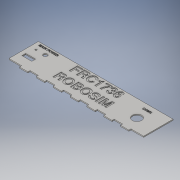
# Autodesk Inventor part: front
Saved by Autodesk Inventor 2016 (Build 200138000, 138)
## iProperties
Created: 2015-08-25
Part Number: front
Material: Generic
Document SubType Name: Modeling
Designer: Chris Gerth
Density: 1 g/cm^3
Appearance: Default
Author: Chris Gerth
Autodesk Inventor part; units mm, degrees
ref_plane "YZ Plane" through (0, 0, 0) normal (1, 0, 0) x (0, 1, 0)
ref_plane "XZ Plane" through (0, 0, 0) normal (0, 1, 0) x (-1, 0, 0)
ref_plane "XY Plane" through (0, 0, 0) normal (0, 0, 1) x (1, 0, 0)
sketch "Sketch1" plane through (0, 0, 0) normal (0, 1, 0) x (-1, 0, 0)
  line L0 (203.2, 31.75) -> (-203.2, 31.75)
  line L1 (-203.2, 31.75) -> (-203.2, -57.15)
  line L2 (-203.2, -57.15) -> (203.2, -57.15)
  line L3 (203.2, -57.15) -> (203.2, 31.75)
  point P0 (0, 0)
  dimension "d0" = 406.4
  dimension "d1" = 88.9
  constraints: 8 end point, 2 parallel, 1 horizontal, 1 perpendicular
  measures "d0" distance of L2.end L1.end
  measures "d1" distance of L1.end L0.end
extrude "Extrusion1" add sketch "Sketch1" along normal blind 3.175
sketch "Sketch2" plane through (0, 3.175, 0) normal (0, 1, 0) x (1, 0, 0)
  line L0 (-203.2, -31.75) -> (203.2, -31.75) projected
  line L1 (-165.1, -31.75) -> (-139.7, -31.75)
  line L2 (-139.7, -31.75) -> (-139.7, -38.1)
  line L3 (-139.7, -38.1) -> (-165.1, -38.1)
  line L4 (-165.1, -38.1) -> (-165.1, -31.75)
  line L5 (-114.3, -31.75) -> (-88.9, -31.75)
  line L6 (-88.9, -31.75) -> (-88.9, -38.1)
  line L7 (-88.9, -38.1) -> (-114.3, -38.1)
  line L8 (-114.3, -38.1) -> (-114.3, -31.75)
  line L9 (-63.5, -31.75) -> (-38.1, -31.75)
  line L10 (-38.1, -31.75) -> (-38.1, -38.1)
  line L11 (-38.1, -38.1) -> (-63.5, -38.1)
  line L12 (-63.5, -38.1) -> (-63.5, -31.75)
  line L13 (-12.7, -31.75) -> (12.7, -31.75)
  line L14 (12.7, -31.75) -> (12.7, -38.1)
  line L15 (12.7, -38.1) -> (-12.7, -38.1)
  line L16 (-12.7, -38.1) -> (-12.7, -31.75)
  line L17 (38.1, -31.75) -> (63.5, -31.75)
  line L18 (63.5, -31.75) -> (63.5, -38.1)
  line L19 (63.5, -38.1) -> (38.1, -38.1)
  line L20 (38.1, -38.1) -> (38.1, -31.75)
  line L21 (88.9, -31.75) -> (114.3, -31.75)
  line L22 (114.3, -31.75) -> (114.3, -38.1)
  line L23 (114.3, -38.1) -> (88.9, -38.1)
  line L24 (88.9, -38.1) -> (88.9, -31.75)
  line L25 (139.7, -31.75) -> (165.1, -31.75)
  line L26 (165.1, -31.75) -> (165.1, -38.1)
  line L27 (165.1, -38.1) -> (139.7, -38.1)
  line L28 (139.7, -38.1) -> (139.7, -31.75)
  point P0 (0, 0)
  dimension "d6" = 50.8
  constraints: 56 end point, 2 horizontal, 2 parallel, 1 collinear, 1 perpendicular, 1 point on line, 47 other
  measures "d6" distance of L1.start L5.start
extrude "Extrusion2" add sketch "Sketch2" against normal blind 3.175
sketch "Sketch3" plane through (-210.3014, 3.175, 39.6064) normal (0, 1, 0) x (1, 0, 0)
  circle A0 centre (355.6026, 45.722) radius 13.97
  point P0 (203.2, 0)
  dimension "d13" = 27.94
  constraints: 1 centre point
  measures "d13" diameter of A0
extrude "Extrusion3" cut sketch "Sketch3" against normal blind 5
sketch "Sketch4" plane through (-216.1175, 3.175, 42.2546) normal (0, 1, 0) x (1, 0, 0)
  line L0 (344.7979, 86.0656) -> (387.5444, 86.0656) construction
  line L1 (387.5444, 86.0656) -> (387.5444, 74.2339) construction
  line L2 (387.5444, 74.2339) -> (344.7979, 74.2339) construction
  line L3 (344.7979, 74.2339) -> (344.7979, 86.0656) construction
  spline S0 degree 2 poles (350.7726, 81.7796) (350.6492, 80.5846) (349.8641, 79.9773) knots 0 0 0 1 1 1
  spline S1 degree 2 poles (349.8641, 79.9773) (349.1431, 79.4193) (347.963, 79.4193) knots 0 0 0 1 1 1
  spline S2 degree 2 poles (347.963, 79.4193) (346.6742, 79.4193) (345.1781, 81.2315) (345.1781, 82.7819) knots 0 0 0 1 2 2 2
  spline S3 degree 2 poles (345.1781, 82.7819) (345.1781, 84.2188) (345.9188, 85.1175) knots 0 0 0 1 1 1
  spline S4 degree 2 poles (345.9188, 85.1175) (346.7039, 86.0656) (348.0865, 86.0656) knots 0 0 0 1 1 1
  spline S5 degree 2 poles (348.0865, 86.0656) (349.2468, 86.0656) (350.743, 84.8212) (350.7726, 83.809) knots 0 0 0 1 2 2 2
  line L4 (350.7726, 83.809) -> (349.5233, 83.809)
  spline S6 degree 2 poles (349.5233, 83.809) (349.474, 84.3126) (348.679, 84.9743) (348.126, 84.9743) knots 0 0 0 1 2 2 2
  spline S7 degree 2 poles (348.126, 84.9743) (347.3507, 84.9743) (346.452, 83.7744) (346.452, 82.7474) knots 0 0 0 1 2 2 2
  spline S8 degree 2 poles (346.452, 82.7474) (346.452, 81.7302) (347.3408, 80.5352) (348.0815, 80.5352) knots 0 0 0 1 2 2 2
  spline S9 degree 2 poles (348.0815, 80.5352) (348.6642, 80.5352) (349.4838, 81.2216) (349.5085, 81.7796) knots 0 0 0 1 2 2 2
  line L5 (349.5085, 81.7796) -> (350.7726, 81.7796)
  spline S10 degree 2 poles (357.5473, 82.7276) (357.5473, 81.2315) (355.8487, 79.4193) (354.4908, 79.4193) knots 0 0 0 1 2 2 2
  spline S11 degree 2 poles (354.4908, 79.4193) (353.0341, 79.4193) (352.2095, 80.4019) knots 0 0 0 1 1 1
  spline S12 degree 2 poles (352.2095, 80.4019) (351.4343, 81.3105) (351.4343, 82.7474) knots 0 0 0 1 1 1
  spline S13 degree 2 poles (351.4343, 82.7474) (351.4343, 84.1299) (352.1651, 85.0385) knots 0 0 0 1 1 1
  spline S14 degree 2 poles (352.1651, 85.0385) (353.0094, 86.0656) (354.5451, 86.0656) knots 0 0 0 1 1 1
  spline S15 degree 2 poles (354.5451, 86.0656) (355.9622, 86.0656) (356.7819, 85.0829) knots 0 0 0 1 1 1
  spline S16 degree 2 poles (356.7819, 85.0829) (357.5473, 84.1596) (357.5473, 82.7276) knots 0 0 0 1 1 1
  spline S17 degree 2 poles (356.2931, 82.7326) (356.2931, 83.7596) (355.3253, 84.9249) (354.471, 84.9249) knots 0 0 0 1 2 2 2
  spline S18 degree 2 poles (354.471, 84.9249) (353.6464, 84.9249) (352.6885, 83.7645) (352.6885, 82.7671) knots 0 0 0 1 2 2 2
  spline S19 degree 2 poles (352.6885, 82.7671) (352.6885, 81.7302) (353.681, 80.5451) (354.5599, 80.5451) knots 0 0 0 1 2 2 2
  spline S20 degree 2 poles (354.5599, 80.5451) (355.3351, 80.5451) (356.2931, 81.7549) (356.2931, 82.7326) knots 0 0 0 1 2 2 2
  line L6 (364.6182, 79.6119) -> (363.3097, 79.6119)
  line L7 (363.3097, 79.6119) -> (363.3097, 84.7669)
  line L8 (363.3097, 84.7669) -> (362.1838, 79.6119)
  line L9 (362.1838, 79.6119) -> (360.8753, 79.6119)
  line L10 (360.8753, 79.6119) -> (359.7446, 84.7422)
  line L11 (359.7446, 84.7422) -> (359.7446, 79.6119)
  line L12 (359.7446, 79.6119) -> (358.4361, 79.6119)
  line L13 (358.4361, 79.6119) -> (358.4361, 85.9619)
  line L14 (358.4361, 85.9619) -> (360.3519, 85.9619)
  line L15 (360.3519, 85.9619) -> (361.5271, 81.1031)
  line L16 (361.5271, 81.1031) -> (362.7171, 85.9619)
  line L17 (362.7171, 85.9619) -> (364.6182, 85.9619)
  line L18 (364.6182, 85.9619) -> (364.6182, 79.6119)
  spline S21 degree 2 poles (370.6324, 81.4833) (370.6324, 80.4908) (369.2301, 79.4094) (367.966, 79.4094) knots 0 0 0 1 2 2 2
  spline S22 degree 2 poles (367.966, 79.4094) (366.8254, 79.4094) (365.502, 80.5056) (365.3983, 81.4932) knots 0 0 0 1 2 2 2
  line L19 (365.3983, 81.4932) -> (366.6624, 81.4932)
  spline S23 degree 2 poles (366.6624, 81.4932) (366.8007, 80.4612) (368.0796, 80.4612) knots 0 0 0 1 1 1
  spline S24 degree 2 poles (368.0796, 80.4612) (368.6721, 80.4612) (369.3782, 80.9056) (369.3782, 81.2907) knots 0 0 0 1 2 2 2
  spline S25 degree 2 poles (369.3782, 81.2907) (369.3782, 81.9968) (368.4993, 82.1647) knots 0 0 0 1 1 1
  line L20 (368.4993, 82.1647) -> (366.9488, 82.461)
  spline S26 degree 2 poles (366.9488, 82.461) (366.3118, 82.5844) (365.5119, 83.4732) (365.5119, 84.0707) knots 0 0 0 1 2 2 2
  spline S27 degree 2 poles (365.5119, 84.0707) (365.5119, 85.0039) (366.7908, 86.0656) (367.9067, 86.0656) knots 0 0 0 1 2 2 2
  spline S28 degree 2 poles (367.9067, 86.0656) (369.1066, 86.0656) (370.4398, 85.0039) (370.4349, 84.0263) knots 0 0 0 1 2 2 2
  line L21 (370.4349, 84.0263) -> (369.2153, 84.0263)
  spline S29 degree 2 poles (369.2153, 84.0263) (369.1856, 84.4904) (368.4499, 85.0286) (367.8574, 85.0286) knots 0 0 0 1 2 2 2
  spline S30 degree 2 poles (367.8574, 85.0286) (366.7414, 85.0286) (366.7414, 84.2089) knots 0 0 0 1 1 1
  spline S31 degree 2 poles (366.7414, 84.2089) (366.7414, 83.6806) (367.4969, 83.5226) knots 0 0 0 1 1 1
  line L22 (367.4969, 83.5226) -> (368.84, 83.2461)
  spline S32 degree 2 poles (368.84, 83.2461) (369.7535, 83.0535) (370.1436, 82.7227) knots 0 0 0 1 1 1
  spline S33 degree 2 poles (370.1436, 82.7227) (370.6324, 82.303) (370.6324, 81.4833) knots 0 0 0 1 1 1
  point P0 (203.2, 0)
  constraints: 2 other
extrude "Extrusion4" cut sketch "Sketch4" against normal blind 1.905
sketch "Sketch5" plane through (-208.4957, 3.175, 40.5353) normal (0, 1, 0) x (1, 0, 0)
  line L0 (17.4181, 47.0558) -> (47.4181, 47.0558)
  line L1 (47.4181, 47.0558) -> (47.4181, 35.5558)
  line L2 (47.4181, 35.5558) -> (17.4181, 35.5558)
  line L3 (17.4181, 35.5558) -> (17.4181, 47.0558)
  point P0 (203.2, 0)
  dimension "d21" = 30
  dimension "d22" = 11.5
  constraints: 8 end point, 2 parallel, 1 horizontal, 1 perpendicular
  measures "d21" distance of L1.end L2.end
  measures "d22" distance of L0.end L1.end
extrude "Extrusion5" cut sketch "Sketch5" against normal blind 5
sketch "Sketch6" plane through (-204.3689, 3.175, 34.8523) normal (0, 1, 0) x (1, 0, 0)
  circle A0 centre (19.1442, 66.6446) radius 2.5
  circle A1 centre (47.3951, 66.6446) radius 6
  point P0 (203.2, 0)
  dimension "d28" = 5
  dimension "d27" = 12
  constraints: 2 centre point
  measures "d28" diameter of A0
  measures "d27" diameter of A1
extrude "Extrusion6" cut sketch "Sketch6" against normal blind 5
sketch "Sketch7" plane through (-201.7656, 3.175, 34.3855) normal (0, 1, 0) x (1, 0, 0)
  line L0 (8.5764, 86.8624) -> (71.354, 86.8624) construction
  line L1 (71.354, 86.8624) -> (71.354, 63.658) construction
  line L2 (71.354, 63.658) -> (8.5764, 63.658) construction
  line L3 (8.5764, 63.658) -> (8.5764, 86.8624) construction
  line L4 (15.3313, 80.4087) -> (14.0227, 80.4087)
  line L5 (14.0227, 80.4087) -> (14.0227, 85.5637)
  line L6 (14.0227, 85.5637) -> (12.8969, 80.4087)
  line L7 (12.8969, 80.4087) -> (11.5884, 80.4087)
  line L8 (11.5884, 80.4087) -> (10.4577, 85.539)
  line L9 (10.4577, 85.539) -> (10.4577, 80.4087)
  line L10 (10.4577, 80.4087) -> (9.1491, 80.4087)
  line L11 (9.1491, 80.4087) -> (9.1491, 86.7587)
  line L12 (9.1491, 86.7587) -> (11.065, 86.7587)
  line L13 (11.065, 86.7587) -> (12.2402, 81.8999)
  line L14 (12.2402, 81.8999) -> (13.4302, 86.7587)
  line L15 (13.4302, 86.7587) -> (15.3313, 86.7587)
  line L16 (15.3313, 86.7587) -> (15.3313, 80.4087)
  line L17 (21.9528, 80.4087) -> (20.6246, 80.4087)
  line L18 (20.6246, 80.4087) -> (20.1752, 81.6826)
  line L19 (20.1752, 81.6826) -> (17.8248, 81.6826)
  line L20 (17.8248, 81.6826) -> (17.3903, 80.4087)
  line L21 (17.3903, 80.4087) -> (16.0571, 80.4087)
  line L22 (16.0571, 80.4087) -> (18.2692, 86.7587)
  line L23 (18.2692, 86.7587) -> (19.7753, 86.7587)
  line L24 (19.7753, 86.7587) -> (21.9528, 80.4087)
  line L25 (19.8642, 82.7739) -> (19.0297, 85.2428)
  line L26 (19.0297, 85.2428) -> (18.2446, 82.7739)
  line L27 (18.2446, 82.7739) -> (19.8642, 82.7739)
  line L28 (23.9823, 80.4087) -> (22.6738, 80.4087)
  line L29 (22.6738, 80.4087) -> (22.6738, 86.7587)
  line L30 (22.6738, 86.7587) -> (23.9823, 86.7587)
  line L31 (23.9823, 86.7587) -> (23.9823, 80.4087)
  line L32 (30.2977, 80.4087) -> (29.0089, 80.4087)
  line L33 (29.0089, 80.4087) -> (26.4413, 84.8477)
  line L34 (26.4413, 84.8477) -> (26.4413, 80.4087)
  line L35 (26.4413, 80.4087) -> (25.1328, 80.4087)
  line L36 (25.1328, 80.4087) -> (25.1328, 86.7587)
  line L37 (25.1328, 86.7587) -> (26.4215, 86.7587)
  line L38 (26.4215, 86.7587) -> (28.9892, 82.4035)
  line L39 (28.9892, 82.4035) -> (28.9892, 86.7587)
  line L40 (28.9892, 86.7587) -> (30.2977, 86.7587)
  line L41 (30.2977, 86.7587) -> (30.2977, 80.4087)
  spline S0 degree 2 poles (38.766, 84.7292) (38.766, 83.8503) (37.7192, 82.6751) (37.0427, 82.6751) knots 0 0 0 1 2 2 2
  line L42 (37.0427, 82.6751) -> (35.2207, 82.6751)
  line L43 (35.2207, 82.6751) -> (35.2207, 80.4087)
  line L44 (35.2207, 80.4087) -> (33.9122, 80.4087)
  line L45 (33.9122, 80.4087) -> (33.9122, 86.7587)
  line L46 (33.9122, 86.7587) -> (36.8995, 86.7587)
  spline S1 degree 2 poles (36.8995, 86.7587) (37.8229, 86.7587) (38.766, 85.6773) (38.766, 84.7292) knots 0 0 0 1 2 2 2
  spline S2 degree 2 poles (37.5019, 84.8082) (37.5019, 85.1983) (37.0822, 85.6674) (36.7119, 85.6674) knots 0 0 0 1 2 2 2
  line L47 (36.7119, 85.6674) -> (35.2207, 85.6674)
  line L48 (35.2207, 85.6674) -> (35.2207, 83.7664)
  line L49 (35.2207, 83.7664) -> (36.7465, 83.7664)
  spline S3 degree 2 poles (36.7465, 83.7664) (37.0575, 83.7664) (37.2847, 84.1071) knots 0 0 0 1 1 1
  spline S4 degree 2 poles (37.2847, 84.1071) (37.5019, 84.4181) (37.5019, 84.8082) knots 0 0 0 1 1 1
  spline S5 degree 2 poles (45.5209, 83.5244) (45.5209, 82.0283) (43.8223, 80.2161) (42.4644, 80.2161) knots 0 0 0 1 2 2 2
  spline S6 degree 2 poles (42.4644, 80.2161) (41.0078, 80.2161) (40.1832, 81.1987) knots 0 0 0 1 1 1
  spline S7 degree 2 poles (40.1832, 81.1987) (39.4079, 82.1073) (39.4079, 83.5442) knots 0 0 0 1 1 1
  spline S8 degree 2 poles (39.4079, 83.5442) (39.4079, 84.9267) (40.1387, 85.8353) knots 0 0 0 1 1 1
  spline S9 degree 2 poles (40.1387, 85.8353) (40.9831, 86.8624) (42.5187, 86.8624) knots 0 0 0 1 1 1
  spline S10 degree 2 poles (42.5187, 86.8624) (43.9359, 86.8624) (44.7556, 85.8797) knots 0 0 0 1 1 1
  spline S11 degree 2 poles (44.7556, 85.8797) (45.5209, 84.9564) (45.5209, 83.5244) knots 0 0 0 1 1 1
  spline S12 degree 2 poles (44.2667, 83.5293) (44.2667, 84.5564) (43.2989, 85.7217) (42.4447, 85.7217) knots 0 0 0 1 2 2 2
  spline S13 degree 2 poles (42.4447, 85.7217) (41.6201, 85.7217) (40.6621, 84.5613) (40.6621, 83.5639) knots 0 0 0 1 2 2 2
  spline S14 degree 2 poles (40.6621, 83.5639) (40.6621, 82.527) (41.6546, 81.3419) (42.5336, 81.3419) knots 0 0 0 1 2 2 2
  spline S15 degree 2 poles (42.5336, 81.3419) (43.3088, 81.3419) (44.2667, 82.5517) (44.2667, 83.5293) knots 0 0 0 1 2 2 2
  line L50 (53.9547, 86.7587) -> (52.1771, 80.4087)
  line L51 (52.1771, 80.4087) -> (51.0019, 80.4087)
  line L52 (51.0019, 80.4087) -> (49.9501, 85.2526)
  line L53 (49.9501, 85.2526) -> (48.9033, 80.4087)
  line L54 (48.9033, 80.4087) -> (47.7281, 80.4087)
  line L55 (47.7281, 80.4087) -> (45.9505, 86.7587)
  line L56 (45.9505, 86.7587) -> (47.3331, 86.7587)
  line L57 (47.3331, 86.7587) -> (48.3108, 82.0036)
  line L58 (48.3108, 82.0036) -> (49.2588, 86.7587)
  line L59 (49.2588, 86.7587) -> (50.6463, 86.7587)
  line L60 (50.6463, 86.7587) -> (51.5944, 81.9493)
  line L61 (51.5944, 81.9493) -> (52.5721, 86.7587)
  line L62 (52.5721, 86.7587) -> (53.9547, 86.7587)
  line L63 (59.4899, 80.4087) -> (54.7447, 80.4087)
  line L64 (54.7447, 80.4087) -> (54.7447, 86.7587)
  line L65 (54.7447, 86.7587) -> (59.3418, 86.7587)
  line L66 (59.3418, 86.7587) -> (59.3418, 85.6674)
  line L67 (59.3418, 85.6674) -> (56.0532, 85.6674)
  line L68 (56.0532, 85.6674) -> (56.0532, 84.2256)
  line L69 (56.0532, 84.2256) -> (59.09, 84.2256)
  line L70 (59.09, 84.2256) -> (59.09, 83.1343)
  line L71 (59.09, 83.1343) -> (56.0532, 83.1343)
  line L72 (56.0532, 83.1343) -> (56.0532, 81.4999)
  line L73 (56.0532, 81.4999) -> (59.4899, 81.4999)
  line L74 (59.4899, 81.4999) -> (59.4899, 80.4087)
  line L75 (65.7659, 80.4087) -> (64.3537, 80.4087)
  spline S16 degree 2 poles (64.3537, 80.4087) (64.1808, 80.8629) (64.1808, 81.1395) knots 0 0 0 1 1 1
  line L76 (64.1808, 81.1395) -> (64.1808, 82.0974)
  spline S17 degree 2 poles (64.1808, 82.0974) (64.1808, 82.4825) (64.0673, 82.6554) knots 0 0 0 1 1 1
  spline S18 degree 2 poles (64.0673, 82.6554) (63.9043, 82.9171) (63.4253, 82.9171) knots 0 0 0 1 1 1
  line L77 (63.4253, 82.9171) -> (61.8749, 82.9171)
  line L78 (61.8749, 82.9171) -> (61.8749, 80.4087)
  line L79 (61.8749, 80.4087) -> (60.5664, 80.4087)
  line L80 (60.5664, 80.4087) -> (60.5664, 86.7587)
  line L81 (60.5664, 86.7587) -> (64.1364, 86.7587)
  spline S19 degree 2 poles (64.1364, 86.7587) (64.7289, 86.7587) (65.1635, 86.3587) knots 0 0 0 1 1 1
  spline S20 degree 2 poles (65.1635, 86.3587) (65.6967, 85.8797) (65.6967, 85.0008) knots 0 0 0 1 1 1
  spline S21 degree 2 poles (65.6967, 85.0008) (65.6967, 83.9787) (64.7635, 83.4652) knots 0 0 0 1 1 1
  spline S22 degree 2 poles (64.7635, 83.4652) (65.44, 83.0998) (65.4597, 82.6455) knots 0 0 0 1 1 1
  line L82 (65.4597, 82.6455) -> (65.5288, 81.095)
  spline S23 degree 2 poles (65.5288, 81.095) (65.5387, 80.8086) (65.7659, 80.6506) knots 0 0 0 1 1 1
  line L83 (65.7659, 80.6506) -> (65.7659, 80.4087)
  spline S24 degree 2 poles (64.4524, 84.9218) (64.4524, 85.6674) (63.7019, 85.6674) knots 0 0 0 1 1 1
  line L84 (63.7019, 85.6674) -> (61.8749, 85.6674)
  line L85 (61.8749, 85.6674) -> (61.8749, 84.0083)
  line L86 (61.8749, 84.0083) -> (63.6772, 84.0083)
  spline S25 degree 2 poles (63.6772, 84.0083) (63.9734, 84.0083) (64.4524, 84.5811) (64.4524, 84.9218) knots 0 0 0 1 2 2 2
  point P0 (203.2, 0)
  constraints: 2 other
extrude "Extrusion7" cut sketch "Sketch7" against normal blind 1.905
sketch "Sketch8" plane through (-218.0152, 3.175, 33.7162) normal (0, 1, 0) x (1, 0, 0)
  line L0 (67.968, 86.6448) -> (350.6513, 86.6448) construction
  line L1 (350.6513, 86.6448) -> (350.6513, 3.4424) construction
  line L2 (350.6513, 3.4424) -> (67.968, 3.4424) construction
  line L3 (67.968, 3.4424) -> (67.968, 86.6448) construction
  line L4 (155.152, 81.865) -> (142.5507, 81.865)
  line L5 (142.5507, 81.865) -> (142.5507, 76.0977)
  line L6 (142.5507, 76.0977) -> (153.6509, 76.0977)
  line L7 (153.6509, 76.0977) -> (153.6509, 71.7326)
  line L8 (153.6509, 71.7326) -> (142.5507, 71.7326)
  line L9 (142.5507, 71.7326) -> (142.5507, 60.83)
  line L10 (142.5507, 60.83) -> (137.3167, 60.83)
  line L11 (137.3167, 60.83) -> (137.3167, 86.23)
  line L12 (137.3167, 86.23) -> (155.152, 86.23)
  line L13 (155.152, 86.23) -> (155.152, 81.865)
  line L14 (179.6237, 60.83) -> (173.9748, 60.83)
  spline S0 degree 2 poles (173.9748, 60.83) (173.2835, 62.6471) (173.2835, 63.7532) knots 0 0 0 1 1 1
  line L15 (173.2835, 63.7532) -> (173.2835, 67.5849)
  spline S1 degree 2 poles (173.2835, 67.5849) (173.2835, 69.1255) (172.8293, 69.8168) knots 0 0 0 1 1 1
  spline S2 degree 2 poles (172.8293, 69.8168) (172.1775, 70.8636) (170.2616, 70.8636) knots 0 0 0 1 1 1
  line L16 (170.2616, 70.8636) -> (164.0597, 70.8636)
  line L17 (164.0597, 70.8636) -> (164.0597, 60.83)
  line L18 (164.0597, 60.83) -> (158.8257, 60.83)
  line L19 (158.8257, 60.83) -> (158.8257, 86.23)
  line L20 (158.8257, 86.23) -> (173.1058, 86.23)
  spline S3 degree 2 poles (173.1058, 86.23) (175.4759, 86.23) (177.214, 84.6302) knots 0 0 0 1 1 1
  spline S4 degree 2 poles (177.214, 84.6302) (179.3471, 82.7143) (179.3471, 79.1986) knots 0 0 0 1 1 1
  spline S5 degree 2 poles (179.3471, 79.1986) (179.3471, 75.1101) (175.6142, 73.056) knots 0 0 0 1 1 1
  spline S6 degree 2 poles (175.6142, 73.056) (178.3201, 71.5944) (178.3991, 69.7773) knots 0 0 0 1 1 1
  line L21 (178.3991, 69.7773) -> (178.6756, 63.5754)
  spline S7 degree 2 poles (178.6756, 63.5754) (178.7151, 62.4298) (179.6237, 61.7978) knots 0 0 0 1 1 1
  line L22 (179.6237, 61.7978) -> (179.6237, 60.83)
  spline S8 degree 2 poles (174.3699, 78.8826) (174.3699, 81.865) (171.3677, 81.865) knots 0 0 0 1 1 1
  line L23 (171.3677, 81.865) -> (164.0597, 81.865)
  line L24 (164.0597, 81.865) -> (164.0597, 75.2286)
  line L25 (164.0597, 75.2286) -> (171.2689, 75.2286)
  spline S9 degree 2 poles (171.2689, 75.2286) (172.454, 75.2286) (174.3699, 77.5197) (174.3699, 78.8826) knots 0 0 0 1 2 2 2
  spline S10 degree 2 poles (205.1027, 69.5008) (204.6089, 64.721) (201.4685, 62.2916) knots 0 0 0 1 1 1
  spline S11 degree 2 poles (201.4685, 62.2916) (198.5848, 60.0597) (193.8643, 60.0597) knots 0 0 0 1 1 1
  spline S12 degree 2 poles (193.8643, 60.0597) (188.7092, 60.0597) (182.7246, 67.3084) (182.7246, 73.5103) knots 0 0 0 1 2 2 2
  spline S13 degree 2 poles (182.7246, 73.5103) (182.7246, 79.2578) (185.6873, 82.8526) knots 0 0 0 1 1 1
  spline S14 degree 2 poles (185.6873, 82.8526) (188.8277, 86.6448) (194.358, 86.6448) knots 0 0 0 1 1 1
  spline S15 degree 2 poles (194.358, 86.6448) (198.9996, 86.6448) (204.9842, 81.6675) (205.1027, 77.6185) knots 0 0 0 1 2 2 2
  line L26 (205.1027, 77.6185) -> (200.1056, 77.6185)
  spline S16 degree 2 poles (200.1056, 77.6185) (199.9081, 79.6331) (196.7282, 82.2798) (194.516, 82.2798) knots 0 0 0 1 2 2 2
  spline S17 degree 2 poles (194.516, 82.2798) (191.4151, 82.2798) (187.8204, 77.4802) (187.8204, 73.372) knots 0 0 0 1 2 2 2
  spline S18 degree 2 poles (187.8204, 73.372) (187.8204, 69.3033) (191.3756, 64.5235) (194.3383, 64.5235) knots 0 0 0 1 2 2 2
  spline S19 degree 2 poles (194.3383, 64.5235) (196.6689, 64.5235) (199.9476, 67.2689) (200.0464, 69.5008) knots 0 0 0 1 2 2 2
  line L27 (200.0464, 69.5008) -> (205.1027, 69.5008)
  line L28 (219.5605, 60.83) -> (214.682, 60.83)
  line L29 (214.682, 60.83) -> (214.682, 77.895)
  line L30 (214.682, 77.895) -> (208.7566, 77.895)
  line L31 (208.7566, 77.895) -> (208.7566, 81.0749)
  spline S20 degree 2 poles (208.7566, 81.0749) (212.2723, 81.4305) (213.7734, 82.2008) knots 0 0 0 1 1 1
  spline S21 degree 2 poles (213.7734, 82.2008) (215.5115, 83.1291) (216.4596, 85.5387) knots 0 0 0 1 1 1
  line L32 (216.4596, 85.5387) -> (219.5605, 85.5387)
  line L33 (219.5605, 85.5387) -> (219.5605, 60.83)
  spline S22 degree 2 poles (244.131, 81.8057) (237.9291, 74.083) (236.2898, 67.5256) knots 0 0 0 1 1 1
  spline S23 degree 2 poles (236.2898, 67.5256) (235.638, 64.879) (235.2429, 60.83) knots 0 0 0 1 1 1
  line L34 (235.2429, 60.83) -> (230.2657, 60.83)
  spline S24 degree 2 poles (230.2657, 60.83) (231.5495, 68.4935) (234.6504, 75.5051) (238.9364, 81.154) knots 0 0 0 1 2 2 2
  line L35 (238.9364, 81.154) -> (226.7499, 81.154)
  line L36 (226.7499, 81.154) -> (226.7499, 85.5387)
  line L37 (226.7499, 85.5387) -> (244.131, 85.5387)
  line L38 (244.131, 85.5387) -> (244.131, 81.8057)
  spline S25 degree 2 poles (263.1513, 67.9009) (263.1513, 64.2865) (258.4111, 60.0005) (254.4411, 60.0005) knots 0 0 0 1 2 2 2
  spline S26 degree 2 poles (254.4411, 60.0005) (251.1229, 60.0005) (248.891, 61.7386) knots 0 0 0 1 1 1
  spline S27 degree 2 poles (248.891, 61.7386) (246.1456, 63.8914) (246.1456, 68.0787) knots 0 0 0 1 1 1
  line L39 (246.1456, 68.0787) -> (250.8859, 68.0787)
  spline S28 degree 2 poles (250.8859, 68.0787) (250.7081, 65.9258) (252.1499, 64.7802) knots 0 0 0 1 1 1
  spline S29 degree 2 poles (252.1499, 64.7802) (253.256, 63.8717) (254.8559, 63.8717) knots 0 0 0 1 1 1
  spline S30 degree 2 poles (254.8559, 63.8717) (256.1594, 63.8717) (258.2136, 66.5578) (258.2136, 68.0589) knots 0 0 0 1 2 2 2
  spline S31 degree 2 poles (258.2136, 68.0589) (258.2136, 69.955) (255.2509, 72.0289) (252.703, 71.9104) knots 0 0 0 1 2 2 2
  line L40 (252.703, 71.9104) -> (252.703, 75.2286)
  spline S32 degree 2 poles (252.703, 75.2286) (257.6408, 75.0903) (257.6408, 78.9813) knots 0 0 0 1 1 1
  spline S33 degree 2 poles (257.6408, 78.9813) (257.6408, 82.2205) (254.2238, 82.2205) knots 0 0 0 1 1 1
  spline S34 degree 2 poles (254.2238, 82.2205) (252.703, 82.2205) (251.9919, 81.4502) knots 0 0 0 1 1 1
  spline S35 degree 2 poles (251.9919, 81.4502) (251.0834, 80.4429) (250.9846, 77.7568) knots 0 0 0 1 1 1
  line L41 (250.9846, 77.7568) -> (246.5209, 77.7568)
  spline S36 degree 2 poles (246.5209, 77.7568) (246.4616, 78.3098) (246.4616, 78.8431) knots 0 0 0 1 1 1
  spline S37 degree 2 poles (246.4616, 78.8431) (246.4616, 82.0428) (251.0241, 86.0917) (254.5003, 86.0917) knots 0 0 0 1 2 2 2
  spline S38 degree 2 poles (254.5003, 86.0917) (257.9963, 86.0917) (260.0702, 84.4524) knots 0 0 0 1 1 1
  spline S39 degree 2 poles (260.0702, 84.4524) (262.3415, 82.7143) (262.3415, 79.4751) knots 0 0 0 1 1 1
  spline S40 degree 2 poles (262.3415, 79.4751) (262.3415, 77.5987) (261.7095, 76.4334) knots 0 0 0 1 1 1
  spline S41 degree 2 poles (261.7095, 76.4334) (261.196, 75.5446) (259.6356, 74.083) knots 0 0 0 1 1 1
  spline S42 degree 2 poles (259.6356, 74.083) (263.1513, 71.8116) (263.1513, 67.9009) knots 0 0 0 1 1 1
  spline S43 degree 2 poles (282.547, 69.0267) (282.547, 65.0765) (280.3151, 62.5681) knots 0 0 0 1 1 1
  spline S44 degree 2 poles (280.3151, 62.5681) (277.9845, 60.0005) (274.1132, 60.0005) knots 0 0 0 1 1 1
  spline S45 degree 2 poles (274.1132, 60.0005) (268.7804, 60.0005) (266.8646, 64.9382) knots 0 0 0 1 1 1
  spline S46 degree 2 poles (266.8646, 64.9382) (265.6202, 68.1577) (265.6202, 74.5966) knots 0 0 0 1 1 1
  spline S47 degree 2 poles (265.6202, 74.5966) (265.6202, 79.5344) (267.9114, 82.7143) knots 0 0 0 1 1 1
  spline S48 degree 2 poles (267.9114, 82.7143) (270.3605, 86.0917) (274.5478, 86.0917) knots 0 0 0 1 1 1
  spline S49 degree 2 poles (274.5478, 86.0917) (277.8067, 86.0917) (281.9347, 82.7933) (282.1322, 79.9294) knots 0 0 0 1 2 2 2
  line L42 (282.1322, 79.9294) -> (277.6487, 79.9294)
  spline S50 degree 2 poles (277.6487, 79.9294) (276.7994, 82.181) (274.3305, 82.181) knots 0 0 0 1 1 1
  spline S51 degree 2 poles (274.3305, 82.181) (272.5529, 82.181) (270.3605, 79.2973) (270.3605, 76.9667) knots 0 0 0 1 2 2 2
  spline S52 degree 2 poles (270.3605, 76.9667) (270.3605, 76.1569) (270.4988, 75.2879) knots 0 0 0 1 1 1
  spline S53 degree 2 poles (270.4988, 75.2879) (272.7307, 77.2037) (274.7848, 77.2037) knots 0 0 0 1 1 1
  spline S54 degree 2 poles (274.7848, 77.2037) (278.3992, 77.2037) (282.547, 73.0165) (282.547, 69.0267) knots 0 0 0 1 2 2 2
  spline S55 degree 2 poles (277.945, 69.165) (277.945, 71.1796) (276.0489, 73.4115) (274.3898, 73.4115) knots 0 0 0 1 2 2 2
  spline S56 degree 2 poles (274.3898, 73.4115) (272.6714, 73.4115) (270.3605, 70.7253) (270.3605, 68.4935) knots 0 0 0 1 2 2 2
  spline S57 degree 2 poles (270.3605, 68.4935) (270.3605, 66.6566) (272.4541, 64.1087) (274.0145, 64.1087) knots 0 0 0 1 2 2 2
  spline S58 degree 2 poles (274.0145, 64.1087) (275.8118, 64.1087) (277.945, 66.8936) (277.945, 69.165) knots 0 0 0 1 2 2 2
  line L43 (149.6611, 19.9611) -> (144.0123, 19.9611)
  spline S59 degree 2 poles (144.0123, 19.9611) (143.321, 21.7782) (143.321, 22.8843) knots 0 0 0 1 1 1
  line L44 (143.321, 22.8843) -> (143.321, 26.716)
  spline S60 degree 2 poles (143.321, 26.716) (143.321, 28.2566) (142.8667, 28.9479) knots 0 0 0 1 1 1
  spline S61 degree 2 poles (142.8667, 28.9479) (142.215, 29.9947) (140.2991, 29.9947) knots 0 0 0 1 1 1
  line L45 (140.2991, 29.9947) -> (134.0972, 29.9947)
  line L46 (134.0972, 29.9947) -> (134.0972, 19.9611)
  line L47 (134.0972, 19.9611) -> (128.8632, 19.9611)
  line L48 (128.8632, 19.9611) -> (128.8632, 45.3611)
  line L49 (128.8632, 45.3611) -> (143.1433, 45.3611)
  spline S62 degree 2 poles (143.1433, 45.3611) (145.5134, 45.3611) (147.2515, 43.7613) knots 0 0 0 1 1 1
  spline S63 degree 2 poles (147.2515, 43.7613) (149.3846, 41.8454) (149.3846, 38.3297) knots 0 0 0 1 1 1
  spline S64 degree 2 poles (149.3846, 38.3297) (149.3846, 34.2412) (145.6517, 32.1871) knots 0 0 0 1 1 1
  spline S65 degree 2 poles (145.6517, 32.1871) (148.3576, 30.7255) (148.4366, 28.9084) knots 0 0 0 1 1 1
  line L50 (148.4366, 28.9084) -> (148.7131, 22.7065)
  spline S66 degree 2 poles (148.7131, 22.7065) (148.7526, 21.5609) (149.6611, 20.9289) knots 0 0 0 1 1 1
  line L51 (149.6611, 20.9289) -> (149.6611, 19.9611)
  spline S67 degree 2 poles (144.4073, 38.0137) (144.4073, 40.9961) (141.4052, 40.9961) knots 0 0 0 1 1 1
  line L52 (141.4052, 40.9961) -> (134.0972, 40.9961)
  line L53 (134.0972, 40.9961) -> (134.0972, 34.3597)
  line L54 (134.0972, 34.3597) -> (141.3064, 34.3597)
  spline S68 degree 2 poles (141.3064, 34.3597) (142.4915, 34.3597) (144.4073, 36.6508) (144.4073, 38.0137) knots 0 0 0 1 2 2 2
  spline S69 degree 2 poles (177.0758, 32.4241) (177.0758, 26.4395) (170.2814, 19.1908) (164.8498, 19.1908) knots 0 0 0 1 2 2 2
  spline S70 degree 2 poles (164.8498, 19.1908) (159.0232, 19.1908) (155.7248, 23.1213) knots 0 0 0 1 1 1
  spline S71 degree 2 poles (155.7248, 23.1213) (152.6238, 26.7555) (152.6238, 32.5031) knots 0 0 0 1 1 1
  spline S72 degree 2 poles (152.6238, 32.5031) (152.6238, 38.0334) (155.547, 41.6676) knots 0 0 0 1 1 1
  spline S73 degree 2 poles (155.547, 41.6676) (158.9244, 45.7759) (165.0671, 45.7759) knots 0 0 0 1 1 1
  spline S74 degree 2 poles (165.0671, 45.7759) (170.7356, 45.7759) (174.0143, 41.8454) knots 0 0 0 1 1 1
  spline S75 degree 2 poles (174.0143, 41.8454) (177.0758, 38.1519) (177.0758, 32.4241) knots 0 0 0 1 1 1
  spline S76 degree 2 poles (172.059, 32.4438) (172.059, 36.5521) (168.1877, 41.2134) (164.7708, 41.2134) knots 0 0 0 1 2 2 2
  spline S77 degree 2 poles (164.7708, 41.2134) (161.4723, 41.2134) (157.6406, 36.5718) (157.6406, 32.5821) knots 0 0 0 1 2 2 2
  spline S78 degree 2 poles (157.6406, 32.5821) (157.6406, 28.4344) (161.6106, 23.6941) (165.1263, 23.6941) knots 0 0 0 1 2 2 2
  spline S79 degree 2 poles (165.1263, 23.6941) (168.2272, 23.6941) (172.059, 28.5331) (172.059, 32.4438) knots 0 0 0 1 2 2 2
  spline S80 degree 2 poles (201.4882, 27.3085) (201.4882, 24.2866) (199.4341, 22.2522) knots 0 0 0 1 1 1
  spline S81 degree 2 poles (199.4341, 22.2522) (197.1034, 19.9611) (192.9162, 19.9611) knots 0 0 0 1 1 1
  line L55 (192.9162, 19.9611) -> (181.184, 19.9611)
  line L56 (181.184, 19.9611) -> (181.184, 45.3611)
  line L57 (181.184, 45.3611) -> (192.1854, 45.3611)
  spline S82 degree 2 poles (192.1854, 45.3611) (195.8591, 45.3611) (200.8364, 41.8059) (200.8364, 38.7445) knots 0 0 0 1 2 2 2
  spline S83 degree 2 poles (200.8364, 38.7445) (200.8364, 35.8213) (198.4268, 33.5104) knots 0 0 0 1 1 1
  spline S84 degree 2 poles (198.4268, 33.5104) (201.4882, 31.081) (201.4882, 27.3085) knots 0 0 0 1 1 1
  spline S85 degree 2 poles (196.5109, 27.9011) (196.5109, 30.9033) (193.094, 30.9033) knots 0 0 0 1 1 1
  line L58 (193.094, 30.9033) -> (186.4181, 30.9033)
  line L59 (186.4181, 30.9033) -> (186.4181, 24.3261)
  line L60 (186.4181, 24.3261) -> (193.094, 24.3261)
  spline S86 degree 2 poles (193.094, 24.3261) (196.5109, 24.3261) (196.5109, 27.9011) knots 0 0 0 1 1 1
  spline S87 degree 2 poles (195.8591, 38.1914) (195.8591, 40.9763) (192.6199, 40.9763) knots 0 0 0 1 1 1
  line L61 (192.6199, 40.9763) -> (186.4181, 40.9763)
  line L62 (186.4181, 40.9763) -> (186.4181, 35.2288)
  line L63 (186.4181, 35.2288) -> (192.4817, 35.2288)
  spline S88 degree 2 poles (192.4817, 35.2288) (195.8591, 35.2288) (195.8591, 38.1914) knots 0 0 0 1 1 1
  spline S89 degree 2 poles (229.3374, 32.4241) (229.3374, 26.4395) (222.5429, 19.1908) (217.1114, 19.1908) knots 0 0 0 1 2 2 2
  spline S90 degree 2 poles (217.1114, 19.1908) (211.2848, 19.1908) (207.9863, 23.1213) knots 0 0 0 1 1 1
  spline S91 degree 2 poles (207.9863, 23.1213) (204.8854, 26.7555) (204.8854, 32.5031) knots 0 0 0 1 1 1
  spline S92 degree 2 poles (204.8854, 32.5031) (204.8854, 38.0334) (207.8086, 41.6676) knots 0 0 0 1 1 1
  spline S93 degree 2 poles (207.8086, 41.6676) (211.186, 45.7759) (217.3286, 45.7759) knots 0 0 0 1 1 1
  spline S94 degree 2 poles (217.3286, 45.7759) (222.9972, 45.7759) (226.2759, 41.8454) knots 0 0 0 1 1 1
  spline S95 degree 2 poles (226.2759, 41.8454) (229.3374, 38.1519) (229.3374, 32.4241) knots 0 0 0 1 1 1
  spline S96 degree 2 poles (224.3206, 32.4438) (224.3206, 36.5521) (220.4493, 41.2134) (217.0324, 41.2134) knots 0 0 0 1 2 2 2
  spline S97 degree 2 poles (217.0324, 41.2134) (213.7339, 41.2134) (209.9022, 36.5718) (209.9022, 32.5821) knots 0 0 0 1 2 2 2
  spline S98 degree 2 poles (209.9022, 32.5821) (209.9022, 28.4344) (213.8722, 23.6941) (217.3879, 23.6941) knots 0 0 0 1 2 2 2
  spline S99 degree 2 poles (217.3879, 23.6941) (220.4888, 23.6941) (224.3206, 28.5331) (224.3206, 32.4438) knots 0 0 0 1 2 2 2
  spline S100 degree 2 poles (252.6635, 27.4468) (252.6635, 23.4768) (247.0541, 19.1513) (241.9978, 19.1513) knots 0 0 0 1 2 2 2
  spline S101 degree 2 poles (241.9978, 19.1513) (237.4353, 19.1513) (232.142, 23.5361) (231.7272, 27.4863) knots 0 0 0 1 2 2 2
  line L64 (231.7272, 27.4863) -> (236.7835, 27.4863)
  spline S102 degree 2 poles (236.7835, 27.4863) (237.3366, 23.3583) (242.4521, 23.3583) knots 0 0 0 1 1 1
  spline S103 degree 2 poles (242.4521, 23.3583) (244.8223, 23.3583) (247.6467, 25.1359) (247.6467, 26.6765) knots 0 0 0 1 2 2 2
  spline S104 degree 2 poles (247.6467, 26.6765) (247.6467, 29.5009) (244.131, 30.1725) knots 0 0 0 1 1 1
  line L65 (244.131, 30.1725) -> (237.9291, 31.3575)
  spline S105 degree 2 poles (237.9291, 31.3575) (235.3812, 31.8513) (232.1815, 35.4065) (232.1815, 37.7964) knots 0 0 0 1 2 2 2
  spline S106 degree 2 poles (232.1815, 37.7964) (232.1815, 41.5294) (237.2971, 45.7759) (241.7608, 45.7759) knots 0 0 0 1 2 2 2
  spline S107 degree 2 poles (241.7608, 45.7759) (246.5604, 45.7759) (251.8932, 41.5294) (251.8734, 37.6186) knots 0 0 0 1 2 2 2
  line L66 (251.8734, 37.6186) -> (246.9949, 37.6186)
  spline S108 degree 2 poles (246.9949, 37.6186) (246.8764, 39.4753) (243.9335, 41.6281) (241.5633, 41.6281) knots 0 0 0 1 2 2 2
  spline S109 degree 2 poles (241.5633, 41.6281) (237.0996, 41.6281) (237.0996, 38.3494) knots 0 0 0 1 1 1
  spline S110 degree 2 poles (237.0996, 38.3494) (237.0996, 36.2361) (240.1215, 35.604) knots 0 0 0 1 1 1
  line L67 (240.1215, 35.604) -> (245.4938, 34.498)
  spline S111 degree 2 poles (245.4938, 34.498) (249.1478, 33.7277) (250.7081, 32.4043) knots 0 0 0 1 1 1
  spline S112 degree 2 poles (250.7081, 32.4043) (252.6635, 30.7255) (252.6635, 27.4468) knots 0 0 0 1 1 1
  line L68 (261.2947, 19.9611) -> (256.0607, 19.9611)
  line L69 (256.0607, 19.9611) -> (256.0607, 45.3611)
  line L70 (256.0607, 45.3611) -> (261.2947, 45.3611)
  line L71 (261.2947, 45.3611) -> (261.2947, 19.9611)
  line L72 (290.5462, 19.9611) -> (285.3122, 19.9611)
  line L73 (285.3122, 19.9611) -> (285.3122, 40.5813)
  line L74 (285.3122, 40.5813) -> (280.8089, 19.9611)
  line L75 (280.8089, 19.9611) -> (275.5748, 19.9611)
  line L76 (275.5748, 19.9611) -> (271.0518, 40.4826)
  line L77 (271.0518, 40.4826) -> (271.0518, 19.9611)
  line L78 (271.0518, 19.9611) -> (265.8178, 19.9611)
  line L79 (265.8178, 19.9611) -> (265.8178, 45.3611)
  line L80 (265.8178, 45.3611) -> (273.4812, 45.3611)
  line L81 (273.4812, 45.3611) -> (278.182, 25.926)
  line L82 (278.182, 25.926) -> (282.942, 45.3611)
  line L83 (282.942, 45.3611) -> (290.5462, 45.3611)
  line L84 (290.5462, 45.3611) -> (290.5462, 19.9611)
  point P0 (203.2, 0)
  constraints: 2 other
extrude "Extrusion8" cut sketch "Sketch8" against normal blind 1.905
equation "\"d16\" = d17"
equation "\"d25\" = d26"
equation "\"d31\" = d28"
equation "\"d17\" = 5"
equation "\"d26\" = 5"
body "Solid1"
